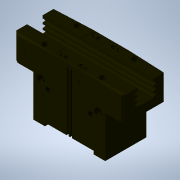
# Autodesk Inventor part: SCHUNK-5524256 Gehaeuse-PGN-plus-P 160-GKS
Saved by Autodesk Inventor 2021 (Build 250183000, 183)
## iProperties
Created: 2025-07-30
Part Number: SCHUNK-5524256 Gehaeuse-PGN-plus-P 160-GKS
Material: Generic
Catalog Web Link: www.cadenas.de
Description: Gehaeuse PGN-plus-P-2-finger parallel gripper
Vendor: SCHUNK
Document SubType Name: Modeling
Designer: psAdmin
Manufacturer: SCHUNK
Mass: 988.597 g
Surface Area: 1168.86 cm^2
Volume: 988.597 cm^3
Density: 1 g/cm^3
Appearance: PSOLRGB-128-128-0
Category: PARTsolutions
Company: SCHUNK
Title: SCHUNK-5524256 Gehaeuse-PGN-plus-P 160-GKS
Author: Cadenas PARTsolutions
Comments: 2-finger parallel gripper
PSOL_IDENT_0: {$CADENAS_DATA/23d-libs/schunk/greifsysteme/greifmodule/greifmodule_pneumatisch/2_finger_parallelgre
PSOL_IDENT_1: ifer/2_finger_universalgreifer/pgn_plus_p/pgnplus_p_geh.prj},238 {VTYP=3D},{NB=SCHUNK-5524256 Gehaeu
PSOL_IDENT_2: se-PGN-plus-P 160-GKS},{LINA=SCHUNK-5524256 Gehaeuse-PGN-plus-P 160-GKS},{NN=Gehaeuse PGN-plus-P},{D
PSOL_IDENT_3: ATE=24.02.2025 16:11:11},{GEOMDATE=14.02.2025 07:59:00},{VERSION=},{LINEID=170},{WBVAR=},{WBNUMERIC=
PSOL_IDENT_4: }  {NB=SCHUNK-5524256 Gehaeuse-PGN-plus-P 160-GKS},{LINA=SCHUNK-5524256 Gehaeuse-PGN-plus-P 160-GKS}
PSOL_IDENT_5: ,{KT=DUMMY},{IDNR=5524256},{TYP=PGN-plus-P 160-GKS},{TYP1=8.000},{TYP2=1.000},{L1=192.000},{B1=72.00
PSOL_IDENT_6: 0},{H1=116.000},{F1=3.500},{WF1=30.000},{L2=125.000},{H2=72.000},{BAVZ=27.390},{TAVZ=86.650},{L1VZ=4
PSOL_IDENT_7: .310},{L2VZ=8.500},{HVZ=5.235},{B1VZ=5.975},{B2VZ=3.170},{F2=0.500},{DNNHS=4.100},{BNNHS=3.400},{LNN
PSOL_IDENT_8: HS=106.600},{L1NNHS=3.000},{L2NNHS=34.100},{LS1=100.000},{LS2=56.000},{SD1=10.500},{ST1=55.500},{G1=
PSOL_IDENT_9: 8.000},{GT1=20.500},{KL1=6.800},{SD2=12.000},{ST2=3.900},{SD3=14.000},{ST3=20.000},{DB1=9.000},{LS3=
PSOL_IDENT_10: 100.000},{LS4=68.000},{B1A=56.000},{B2A=69.000},{RA=6.500},{TA=1.000},{L1TYP=92.000},{L2TYP=15.100},
PSOL_IDENT_11: {LTYP=64.300},{BTYP=16.300},{TTYP=0.700},{B3A=113.100},{B4A=85.100},{T2A=5.500},{R1A=7.450},{R2A=15.
PSOL_IDENT_12: 000},{G2=5.000},{LG1=111.500},{LG2=99.500},{TKT=1.500},{D1=1.000},{D2=0.500},{TT=1.800},{LB1=148.500
PSOL_IDENT_13: },{DB2=8.200},{TB2=86.350},{DB3=6.800},{LD1=0.000},{D3=0.000},{TD3=0.000},{L3=138.500},{H3=55.750},{
PSOL_IDENT_14: B2=20.000},{B3=61.325},{R1=35.000},{H4=30.000},{LG3=58.000},{LG4=74.000},{SD4=0.000},{ST4=0.000},{G3=
PSOL_IDENT_15: 5.000},{TKT2=1.500},{D4=1.000},{D5=0.500},{TT2=1.800},{G4=9.730},{GT4=7.000},{KT4=11.000},{LG5=58.00
PSOL_IDENT_16: 0},{LG6=74.000},{SDZHU=8.000},{TSZHU=2.900},{G5=5.000},{GT5=13.000},{KT5=15.500},{LS5=26.000},{LS6=5
PSOL_IDENT_17: 6.000},{SD5=7.000},{ST5=1.500},{G6=3.000},{GT6=6.000},{KT6=7.500},{SD6=5.000},{ST6=0.600},{LS7=43.00
PSOL_IDENT_18: 0},{LS8=56.000},{H5=50.000},{LG7=86.000},{LG8=45.000},{G7=4.000},{GT7=7.000},{KT7=10.000},{LG9=59.40
PSOL_IDENT_19: 0},{LG10=6.500},{LG11=66.900},{G8=3.000},{GT8=5.000},{KT8=8.000},{L1G=61.000},{HG=6.000},{LA=29.000}
PSOL_IDENT_20: ,{LB=24.000},{LKLH=6.5},{L1DYNFASE=56.000},{FDYNFASE=5.000},{BMMS=0.000},{TMMS=0.000},{LMMS=0.000},{
PSOL_IDENT_21: FASEDYN=0.500},{SLGD=5.0},{SLGT=4.0},{LAGD=5.0},{LAGT=4.0},{CNSCTN=}
NB: SCHUNK-5524256 Gehaeuse-PGN-plus-P 160-GKS
NN: Gehaeuse PGN-plus-P
NT: 2-finger parallel gripper
NBSYN: SCHUNK-$IDNR. Gehaeuse-$TYP.
LINA: SCHUNK-5524256 Gehaeuse-PGN-plus-P 160-GKS
CATALOG: SCHUNK
IDNR: 5524256
TYP: PGN-plus-P 160-GKS
TYP1: 8
TYP2: 1
L1: 192
B1: 72
H1: 116
F1: 3.5
WF1: 30
L2: 125
H2: 72
BAVZ: 27.39
TAVZ: 86.65
L1VZ: 4.31
L2VZ: 8.5
HVZ: 5.235
B1VZ: 5.975
B2VZ: 3.17
F2: 0.5
DNNHS: 4.1
BNNHS: 3.4
LNNHS: 106.6
L1NNHS: 3
L2NNHS: 34.1
LS1: 100
LS2: 56
SD1: 10.5
ST1: 55.5
G1: 8
GT1: 20.5
KL1: 6.8
SD2: 12
ST2: 3.9
SD3: 14
ST3: 20
DB1: 9
LS3: 100
LS4: 68
B1A: 56
B2A: 69
RA: 6.5
TA: 1
L1TYP: 92
L2TYP: 15.1
LTYP: 64.3
BTYP: 16.3
TTYP: 0.7
B3A: 113.1
B4A: 85.1
T2A: 5.5
R1A: 7.45
R2A: 15
G2: 5
LG1: 111.5
LG2: 99.5
TKT: 1.5
D1: 1
D2: 0.5
TT: 1.8
LB1: 148.5
DB2: 8.2
TB2: 86.35
DB3: 6.8
LD1: 0
D3: 0
TD3: 0
L3: 138.5
H3: 55.75
B2: 20
B3: 61.325
R1: 35
H4: 30
LG3: 58
LG4: 74
SD4: 0
ST4: 0
G3: 5
TKT2: 1.5
D4: 1
D5: 0.5
TT2: 1.8
G4: 9.73
GT4: 7
KT4: 11
LG5: 58
LG6: 74
SDZHU: 8
TSZHU: 2.9
G5: 5
GT5: 13
KT5: 15.5
LS5: 26
LS6: 56
SD5: 7
ST5: 1.5
G6: 3
GT6: 6
KT6: 7.5
SD6: 5
ST6: 0.6
LS7: 43
LS8: 56
H5: 50
LG7: 86
LG8: 45
G7: 4
GT7: 7
KT7: 10
LG9: 59.4
LG10: 6.5
LG11: 66.9
G8: 3
GT8: 5
KT8: 8
L1G: 61
HG: 6
LA: 29
LB: 24
L1DYNFASE: 56
FDYNFASE: 5
BMMS: 0
TMMS: 0
LMMS: 0
FASEDYN: 0.5
SLGD: 5
SLGT: 4
LAGD: 5
LAGT: 4
SUPPLIER: SCHUNK
ARTICLENO: SCHUNK-5524256 Gehaeuse-PGN-plus-P 160-GKS
BOMINFO: SCHUNK-5524256 Gehaeuse-PGN-plus-P 160-GKS
CREATOR: CADENAS GmbH
Autodesk Inventor part; units mm, degrees
ref_plane "YZ Plane" through (0, 0, 0) normal (1, 0, 0) x (0, 1, 0)
ref_plane "XZ Plane" through (0, 0, 0) normal (0, 1, 0) x (-1, 0, 0)
ref_plane "XY Plane" through (0, 0, 0) normal (0, 0, 1) x (1, 0, 0)
sketch "Sketch_1" plane through (0, 0, 0) normal (0, 1, 0) x (-1, 0, 0)
  line L0 (96, -32.5) -> (96, 32.5)
  line L1 (96, 32.5) -> (89.9378, 36)
  line L2 (89.9378, 36) -> (-89.9378, 36)
  line L3 (-89.9378, 36) -> (-96, 32.5)
  line L4 (-96, 32.5) -> (-96, -32.5)
  line L5 (-96, -32.5) -> (-89.9378, -36)
  line L6 (-89.9378, -36) -> (89.9378, -36)
  line L7 (89.9378, -36) -> (96, -32.5)
  constraints: 16 end point
extrude "Extrusion1" add sketch "Sketch_1" along normal blind 116
sketch "Sketch_2" plane through (0, 0, 0) normal (0, 0, 1) x (1, 0, 0)
  line L0 (62.5, 72) -> (62.5, 0)
  line L1 (62.5, 0) -> (96, 0)
  line L2 (96, 0) -> (96, 72)
  line L3 (96, 72) -> (62.5, 72)
  constraints: 8 end point
extrude "Extrusion2" cut sketch "Sketch_2" along normal mid plane 72
sketch "Sketch_3" plane through (0, 0, 0) normal (0, 0, 1) x (1, 0, 0)
  line L0 (-96, 0) -> (-62.5, 0)
  line L1 (-62.5, 0) -> (-62.5, 72)
  line L2 (-62.5, 72) -> (-96, 72)
  line L3 (-96, 72) -> (-96, 0)
  constraints: 8 end point
extrude "Extrusion3" cut sketch "Sketch_3" along normal mid plane 72
sketch "Sketch_4" plane through (0, 0, 0) normal (1, 0, 0) x (0, 1, 0)
  line L0 (116, 13.695) -> (86.65, 13.695)
  line L1 (86.65, 13.695) -> (86.65, -13.695)
  line L2 (86.65, -13.695) -> (116, -13.695)
  line L3 (116, -13.695) -> (116, 13.695)
  constraints: 8 end point
extrude "Extrusion4" cut sketch "Sketch_4" along normal mid plane 192
sketch "Sketch_5" plane through (0, 0, 0) normal (1, 0, 0) x (0, 1, 0)
  line L0 (92.3915, 18.93) -> (89.5285, 18.93)
  arc A0 (89.5285, 18.93) -> (89.3353, 18.7818) centre (89.5285, 18.73) ccw
  line L1 (89.3353, 18.7818) -> (88.0122, 13.8432)
  arc A1 (87.819, 13.695) -> (88.0122, 13.8432) centre (87.819, 13.895) ccw
  line L2 (87.819, 13.695) -> (94.101, 13.695)
  arc A2 (93.9078, 13.8432) -> (94.101, 13.695) centre (94.101, 13.895) ccw
  line L3 (93.9078, 13.8432) -> (92.5847, 18.7818)
  arc A3 (92.5847, 18.7818) -> (92.3915, 18.93) centre (92.3915, 18.73) ccw
  constraints: 8 end point, 8 point on circle, 4 centre point
extrude "Extrusion5" cut sketch "Sketch_5" along normal mid plane 192
pattern_linear "Rectangular Pattern1" count 3 spacing 8.5 along (0, 1, 0) of "Extrusion5"
sketch "Sketch_7" plane through (0, 0, 0) normal (1, 0, 0) x (0, 1, 0)
  line L0 (94.101, -13.695) -> (87.819, -13.695)
  arc A0 (88.0122, -13.8432) -> (87.819, -13.695) centre (87.819, -13.895) ccw
  line L1 (88.0122, -13.8432) -> (89.3353, -18.7818)
  arc A1 (89.3353, -18.7818) -> (89.5285, -18.93) centre (89.5285, -18.73) ccw
  line L2 (89.5285, -18.93) -> (92.3915, -18.93)
  arc A2 (92.3915, -18.93) -> (92.5847, -18.7818) centre (92.3915, -18.73) ccw
  line L3 (92.5847, -18.7818) -> (93.9078, -13.8432)
  arc A3 (94.101, -13.695) -> (93.9078, -13.8432) centre (94.101, -13.895) ccw
  constraints: 8 end point, 8 point on circle, 4 centre point
extrude "Extrusion6" cut sketch "Sketch_7" along normal mid plane 192
pattern_linear "Rectangular Pattern2" count 3 spacing 8.5 along (0, 1, 0) of "Extrusion6"
sketch "Sketch_9" plane through (0, 0, 0) normal (1, 0, 0) x (0, 1, 0)
  line L0 (116, -35.5) -> (115.5, -36)
  line L1 (115.5, -36) -> (116, -36)
  line L2 (116, -36) -> (116, -35.5)
  constraints: 6 end point
extrude "Extrusion7" cut sketch "Sketch_9" along normal mid plane 192
sketch "Sketch_10" plane through (0, 0, 0) normal (1, 0, 0) x (0, 1, 0)
  line L0 (116, 36) -> (115.5, 36)
  line L1 (115.5, 36) -> (116, 35.5)
  line L2 (116, 35.5) -> (116, 36)
  constraints: 6 end point
extrude "Extrusion8" cut sketch "Sketch_10" along normal mid plane 192
sketch "Sketch_36" plane through (28, 0, 0) normal (1, 0, 0) x (0, 0, -1)
  line L0 (-36, 116) -> (-36, 115.6464)
  line L1 (-36, 115.6464) -> (-35.6464, 116)
  line L2 (-35.6464, 116) -> (-36, 116)
  constraints: 6 end point
sketch "Sketch_93" plane through (96, 0, 0) normal (1, 0, 0) x (0, 0, -1)
  line L0 (-36, 116) -> (-36, 112.4645)
  line L1 (-36, 112.4645) -> (-32.4645, 116)
  line L2 (-32.4645, 116) -> (-36, 116)
  constraints: 6 end point
loft "Loft1" cut profiles "Sketch_36", "Sketch_93"
sketch "Sketch_94" plane through (-28, 0, 0) normal (1, 0, 0) x (0, 0, -1)
  line L0 (-36, 116) -> (-36, 115.6464)
  line L1 (-36, 115.6464) -> (-35.6464, 116)
  line L2 (-35.6464, 116) -> (-36, 116)
  constraints: 6 end point
sketch "Sketch_95" plane through (-96, 0, 0) normal (1, 0, 0) x (0, 0, -1)
  line L0 (-36, 116) -> (-36, 112.4645)
  line L1 (-36, 112.4645) -> (-32.4645, 116)
  line L2 (-32.4645, 116) -> (-36, 116)
  constraints: 6 end point
loft "Loft2" cut profiles "Sketch_95", "Sketch_94"
sketch "Sketch_96" plane through (28, 0, 0) normal (1, 0, 0) x (0, 0, -1)
  line L0 (36, 116) -> (35.6464, 116)
  line L1 (35.6464, 116) -> (36, 115.6464)
  line L2 (36, 115.6464) -> (36, 116)
  constraints: 6 end point
sketch "Sketch_97" plane through (96, 0, 0) normal (1, 0, 0) x (0, 0, -1)
  line L0 (36, 116) -> (32.4645, 116)
  line L1 (32.4645, 116) -> (36, 112.4645)
  line L2 (36, 112.4645) -> (36, 116)
  constraints: 6 end point
loft "Loft3" cut profiles "Sketch_96", "Sketch_97"
sketch "Sketch_98" plane through (-28, 0, 0) normal (1, 0, 0) x (0, 0, -1)
  line L0 (36, 116) -> (35.6464, 116)
  line L1 (35.6464, 116) -> (36, 115.6464)
  line L2 (36, 115.6464) -> (36, 116)
  constraints: 6 end point
sketch "Sketch_99" plane through (-96, 0, 0) normal (1, 0, 0) x (0, 0, -1)
  line L0 (36, 116) -> (32.4645, 116)
  line L1 (32.4645, 116) -> (36, 112.4645)
  line L2 (36, 112.4645) -> (36, 116)
  constraints: 6 end point
loft "Loft4" cut profiles "Sketch_99", "Sketch_98"
sketch "Sketch_11" plane through (0, 0, 0) normal (0, 1, 0) x (-1, 0, 0)
  arc A0 (-4.7, 35.2456) -> (-1.3, 35.2456) centre (-3, 34.1) ccw
  line L0 (-1.3, 35.2456) -> (-1.3, 37)
  line L1 (-1.3, 37) -> (-4.7, 37)
  line L2 (-4.7, 37) -> (-4.7, 35.2456)
  constraints: 6 end point, 2 point on circle, 1 centre point
extrude "Extrusion9" cut sketch "Sketch_11" along normal blind 106.6
pattern_linear "Rectangular Pattern3" count 2 spacing 6 along (-1, 0, 0) of "Extrusion9"
sketch "Sketch_13" plane through (0, 0, 36) normal (0, 0, 1) x (1, 0, 0)
  circle A0 centre (3, 106.6) radius 1.7
  constraints: 1 centre point
extrude "Extrusion10" cut sketch "Sketch_13" against normal blind 2.05
pattern_linear "Rectangular Pattern4" count 2 spacing 6 along (-1, 0, 0) of "Extrusion10"
sketch "Sketch_15" plane through (0, 106.6, 0) normal (0, 1, 0) x (1, 0, 0)
  line L0 (3, -100) -> (3, 100)
  arc A0 (3, -36.15) -> (3, -32.05) centre (3, -34.1) ccw
  line L1 (3, -36.15) -> (3, -32.05)
  constraints: 4 end point, 2 point on circle, 1 centre point
revolve "Revolution1" cut sketch "Sketch_15" angle 360 about axis through (3, 106.6, 100) along (0, 0, 1)
pattern_linear "Rectangular Pattern5" count 2 spacing 6 along (-1, 0, 0) of "Revolution1"
sketch "Sketch_17" plane through (50, 0, 0) normal (1, 0, 0) x (0, 0, -1)
  line L0 (28, 0) -> (28, 116)
  line L1 (28, 116) -> (33.25, 116)
  line L2 (33.25, 116) -> (33.25, 60.5)
  line L3 (33.25, 60.5) -> (31.3235, 60.5)
  line L4 (31.3235, 60.5) -> (31.3235, 0)
  line L5 (31.3235, 0) -> (28, 0)
  line L6 (28, 0) -> (28, 116)
  constraints: 14 end point
revolve "Revolution2" cut sketch "Sketch_17" angle 360 about axis through (50, 0, -28) along (0, -1, 0)
thread "Thread1" size "M8x1.25" class "6H" standard "ISO Metric profile" length 20.5
pattern_linear "Rectangular Pattern6" count 2 spacing 114.6124 along (-0.872506, 0, 0.4886034) of "Revolution2"
sketch "Sketch_108" plane through (50, 0, 0) normal (1, 0, 0) x (0, 0, -1)
  line L0 (28, 0) -> (28, 116)
  line L1 (28, 116) -> (31.4, 116)
  line L2 (31.4, 116) -> (31.4, 0)
  line L3 (31.4, 0) -> (28, 0)
  line L4 (28, 0) -> (28, 116)
  constraints: 10 end point
revolve "Revolution3" cut sketch "Sketch_108" angle 360 about axis through (50, 0, -28) along (0, -1, 0)
pattern_linear "Rectangular Pattern7" count 2 spacing 114.6124 along (-0.872506, 0, 0.4886034) of "Revolution3"
sketch "Sketch_19" plane through (50, 0, 0) normal (1, 0, 0) x (0, 0, -1)
  line L0 (-28, 0) -> (-28, 116)
  line L1 (-28, 116) -> (-22.75, 116)
  line L2 (-22.75, 116) -> (-22.75, 60.5)
  line L3 (-22.75, 60.5) -> (-24.6765, 60.5)
  line L4 (-24.6765, 60.5) -> (-24.6765, 3.9)
  line L5 (-24.6765, 3.9) -> (-22, 3.9)
  line L6 (-22, 3.9) -> (-22, 0)
  line L7 (-22, 0) -> (-28, 0)
  line L8 (-28, 0) -> (-28, 116)
  constraints: 18 end point
revolve "Revolution4" cut sketch "Sketch_19" angle 360 about axis through (50, 0, 28) along (0, -1, 0)
thread "Thread2" size "M8x1.25" class "6H" standard "ISO Metric profile" length 16.6
pattern_linear "Rectangular Pattern8" count 2 spacing 114.6124 along (-0.872506, 0, -0.4886034) of "Revolution4"
sketch "Sketch_110" plane through (50, 0, 0) normal (1, 0, 0) x (0, 0, -1)
  line L0 (-28, 0) -> (-28, 116)
  line L1 (-28, 116) -> (-24.6, 116)
  line L2 (-24.6, 116) -> (-24.6, 0)
  line L3 (-24.6, 0) -> (-28, 0)
  line L4 (-28, 0) -> (-28, 116)
  constraints: 10 end point
revolve "Revolution5" cut sketch "Sketch_110" angle 360 about axis through (50, 0, 28) along (0, -1, 0)
pattern_linear "Rectangular Pattern9" count 2 spacing 114.6124 along (-0.872506, 0, -0.4886034) of "Revolution5"
sketch "Sketch_21" plane through (50, 0, 0) normal (1, 0, 0) x (0, 0, -1)
  line L0 (36, 68) -> (-36, 68)
  line L1 (-36, 68) -> (-36, 75)
  line L2 (-36, 75) -> (-16, 75)
  line L3 (-16, 75) -> (-16, 72.5)
  line L4 (-16, 72.5) -> (32.1, 72.5)
  line L5 (32.1, 72.5) -> (32.1, 74)
  line L6 (32.1, 74) -> (36, 74)
  line L7 (36, 74) -> (36, 68)
  line L8 (36, 68) -> (-36, 68)
  constraints: 18 end point
revolve "Revolution6" cut sketch "Sketch_21" angle 360 about axis through (50, 68, -36) along (0, 0, -1)
pattern_linear "Rectangular Pattern10" count 2 spacing 100 along (-1, 0, 0) of "Revolution6"
sketch "Sketch_23" plane through (0, 116, 0) normal (0, 1, 0) x (1, 0, 0)
  line L0 (-28, 28) -> (-28, -28)
  arc A0 (-28, -28) -> (-21.5, -34.5) centre (-21.5, -28) ccw
  line L1 (-21.5, -34.5) -> (21.5, -34.5)
  arc A1 (21.5, -34.5) -> (28, -28) centre (21.5, -28) ccw
  line L2 (28, -28) -> (28, 28)
  arc A2 (28, 28) -> (21.5, 34.5) centre (21.5, 28) ccw
  line L3 (21.5, 34.5) -> (-21.5, 34.5)
  arc A3 (-21.5, 34.5) -> (-28, 28) centre (-21.5, 28) ccw
  constraints: 8 end point, 8 point on circle, 4 centre point
extrude "Extrusion11" cut sketch "Sketch_23" against normal blind 1
sketch "Sketch_24" plane through (0, 0, 36) normal (0, 0, 1) x (1, 0, 0)
  arc A0 (23.25, 108.3) -> (23.25, 92) centre (23.25, 100.15) ccw
  line L0 (23.25, 92) -> (71.25, 92)
  arc A1 (71.25, 92) -> (71.25, 108.3) centre (71.25, 100.15) ccw
  line L1 (71.25, 108.3) -> (23.25, 108.3)
  constraints: 4 end point, 4 point on circle, 2 centre point
extrude "Extrusion12" cut sketch "Sketch_24" against normal blind 0.7
sketch "Sketch_70" plane through (0, 0, 36) normal (0, 0, 1) x (1, 0, 0)
  arc A0 (-71.25, 108.3) -> (-71.25, 92) centre (-71.25, 100.15) ccw
  line L0 (-71.25, 92) -> (-23.25, 92)
  arc A1 (-23.25, 92) -> (-23.25, 108.3) centre (-23.25, 100.15) ccw
  line L1 (-23.25, 108.3) -> (-71.25, 108.3)
  constraints: 4 end point, 4 point on circle, 2 centre point
extrude "Extrusion13" cut sketch "Sketch_70" against normal blind 0.7
sketch "Sketch_58" plane through (0, 0, 0) normal (0, 1, 0) x (-1, 0, 0)
  line L0 (56.55, -7.201) -> (56.55, 7.201)
  arc A0 (56.55, 7.201) -> (47.1959, 21.0979) centre (41.55, 7.201) ccw
  arc A1 (42.55, 28) -> (47.1959, 21.0979) centre (50, 28) ccw
  line L1 (42.55, 28) -> (42.55, 38)
  line L2 (42.55, 38) -> (-42.55, 38)
  line L3 (-42.55, 38) -> (-42.55, 28)
  arc A2 (-47.1959, 21.0979) -> (-42.55, 28) centre (-50, 28) ccw
  arc A3 (-47.1959, 21.0979) -> (-56.55, 7.201) centre (-41.55, 7.201) ccw
  line L4 (-56.55, 7.201) -> (-56.55, -7.201)
  arc A4 (-56.55, -7.201) -> (-47.1959, -21.0979) centre (-41.55, -7.201) ccw
  arc A5 (-42.55, -28) -> (-47.1959, -21.0979) centre (-50, -28) ccw
  line L5 (-42.55, -28) -> (-42.55, -36)
  line L6 (-42.55, -36) -> (42.55, -36)
  line L7 (42.55, -36) -> (42.55, -28)
  arc A6 (47.1959, -21.0979) -> (42.55, -28) centre (50, -28) ccw
  arc A7 (47.1959, -21.0979) -> (56.55, -7.201) centre (41.55, -7.201) ccw
  constraints: 16 end point, 16 point on circle, 8 centre point
extrude "Extrusion14" cut sketch "Sketch_58" along normal blind 5.5
sketch "Sketch_45" plane through (0, 0, 0) normal (1, 0, 0) x (0, 1, 0)
  line L0 (86, -35.9) -> (86, -36)
  line L1 (86, -36) -> (116, -36)
  line L2 (116, -36) -> (116, -35.9)
  line L3 (116, -35.9) -> (86, -35.9)
  constraints: 8 end point
extrude "Extrusion15" cut sketch "Sketch_45" along normal mid plane 192
sketch "Sketch_54" plane through (0, 0, 0) normal (1, 0, 0) x (0, 1, 0)
  line L0 (50, -35.9) -> (0, -35.9)
  line L1 (0, -35.9) -> (0, -36)
  line L2 (0, -36) -> (50, -36)
  line L3 (50, -36) -> (50, -35.9)
  constraints: 8 end point
extrude "Extrusion16" cut sketch "Sketch_54" along normal mid plane 192
sketch "Sketch_27" plane through (0, 0, 0) normal (1, 0, 0) x (0, 1, 0)
  line L0 (111.5, 35.9) -> (111.5, 36)
  line L1 (111.5, 36) -> (114, 36)
  line L2 (114, 36) -> (114, 35.6)
  line L3 (114, 35.6) -> (113.7, 35.9)
  line L4 (113.7, 35.9) -> (111.5, 35.9)
  line L5 (111.5, 35.9) -> (111.5, 36)
  constraints: 12 end point
revolve "Revolution7" cut sketch "Sketch_27" angle 360 about axis through (0, 111.5, 35.9) along (0, 0, -1)
sketch "Sketch_28" plane through (0, 0, 0) normal (1, 0, 0) x (0, 1, 0)
  line L0 (99.5, -35.9) -> (99.5, -35.8)
  line L1 (99.5, -35.8) -> (101.7, -35.8)
  line L2 (101.7, -35.8) -> (102, -35.5)
  line L3 (102, -35.5) -> (102, -35.9)
  line L4 (102, -35.9) -> (99.5, -35.9)
  line L5 (99.5, -35.9) -> (99.5, -35.8)
  constraints: 12 end point
revolve "Revolution8" cut sketch "Sketch_28" angle 360 about axis through (0, 99.5, -35.9) along (0, 0, -1)
sketch "Sketch_29" plane through (0, 111.5, 35.9) normal (0, 0, 1) x (0, 1, 0)
  arc A0 (-1, 0.866) -> (-1.25, 0.433) centre (-1.125, 0.6495) ccw
  arc A1 (-1.25, -0.433) -> (-1.25, 0.433) centre (-1.5, 0) ccw
  arc A2 (-1.25, -0.433) -> (-1, -0.866) centre (-1.125, -0.6495) ccw
  arc A3 (-0.25, -1.299) -> (-1, -0.866) centre (-0.75, -1.299) ccw
  arc A4 (-0.25, -1.299) -> (0.25, -1.299) centre (0, -1.299) ccw
  arc A5 (1, -0.866) -> (0.25, -1.299) centre (0.75, -1.299) ccw
  arc A6 (1, -0.866) -> (1.25, -0.433) centre (1.125, -0.6495) ccw
  arc A7 (1.25, 0.433) -> (1.25, -0.433) centre (1.5, 0) ccw
  arc A8 (1.25, 0.433) -> (1, 0.866) centre (1.125, 0.6495) ccw
  arc A9 (0.25, 1.299) -> (1, 0.866) centre (0.75, 1.299) ccw
  arc A10 (0.25, 1.299) -> (-0.25, 1.299) centre (0, 1.299) ccw
  arc A11 (-1, 0.866) -> (-0.25, 1.299) centre (-0.75, 1.299) ccw
  constraints: 24 point on circle, 12 centre point
extrude "Extrusion17" cut sketch "Sketch_29" against normal blind 1.8
sketch "Sketch_30" plane through (0, 99.5, -35.8) normal (0, 0, -1) x (0, 1, 0)
  arc A0 (-1, 0.866) -> (-1.25, 0.433) centre (-1.125, 0.6495) ccw
  arc A1 (-1.25, -0.433) -> (-1.25, 0.433) centre (-1.5, 0) ccw
  arc A2 (-1.25, -0.433) -> (-1, -0.866) centre (-1.125, -0.6495) ccw
  arc A3 (-0.25, -1.299) -> (-1, -0.866) centre (-0.75, -1.299) ccw
  arc A4 (-0.25, -1.299) -> (0.25, -1.299) centre (0, -1.299) ccw
  arc A5 (1, -0.866) -> (0.25, -1.299) centre (0.75, -1.299) ccw
  arc A6 (1, -0.866) -> (1.25, -0.433) centre (1.125, -0.6495) ccw
  arc A7 (1.25, 0.433) -> (1.25, -0.433) centre (1.5, 0) ccw
  arc A8 (1.25, 0.433) -> (1, 0.866) centre (1.125, 0.6495) ccw
  arc A9 (0.25, 1.299) -> (1, 0.866) centre (0.75, 1.299) ccw
  arc A10 (0.25, 1.299) -> (-0.25, 1.299) centre (0, 1.299) ccw
  arc A11 (-1, 0.866) -> (-0.25, 1.299) centre (-0.75, 1.299) ccw
  constraints: 24 point on circle, 12 centre point
extrude "Extrusion18" cut sketch "Sketch_30" against normal blind 1.8
sketch "Sketch_31" plane through (0, 0, 0) normal (0, 0, 1) x (1, 0, 0)
  line L0 (74.25, 0) -> (74.25, 86.65)
  line L1 (74.25, 86.65) -> (77.65, 86.65)
  line L2 (77.65, 86.65) -> (77.65, 86.35)
  line L3 (77.65, 86.35) -> (78.35, 86.35)
  line L4 (78.35, 86.35) -> (78.35, 0)
  line L5 (78.35, 0) -> (74.25, 0)
  line L6 (74.25, 0) -> (74.25, 86.65)
  constraints: 14 end point
revolve "Revolution9" cut sketch "Sketch_31" angle 360 about axis through (74.25, 0, 0) along (0, -1, 0)
pattern_linear "Rectangular Pattern11" count 2 spacing 148.5 along (-1, 0, 0) of "Revolution9"
sketch "Sketch_35" plane through (0, 55.75, 0) normal (0, 1, 0) x (1, 0, 0)
  line L0 (62.5, 30.6625) -> (62.5, -30.6625)
  arc A0 (69.25, -10) -> (62.5, -30.6625) centre (97.5, -30.6625) ccw
  line L1 (69.25, -10) -> (69.25, 10)
  arc A1 (62.5, 30.6625) -> (69.25, 10) centre (97.5, 30.6625) ccw
  constraints: 4 end point, 4 point on circle, 2 centre point
extrude "Extrusion19" add sketch "Sketch_35" along normal blind 16.25
sketch "Sketch_92" plane through (0, 55.75, 0) normal (0, 1, 0) x (1, 0, 0)
  line L0 (-69.25, 10) -> (-69.25, -10)
  arc A0 (-62.5, -30.6625) -> (-69.25, -10) centre (-97.5, -30.6625) ccw
  line L1 (-62.5, -30.6625) -> (-62.5, 30.6625)
  arc A1 (-69.25, 10) -> (-62.5, 30.6625) centre (-97.5, 30.6625) ccw
  constraints: 4 end point, 4 point on circle, 2 centre point
extrude "Extrusion20" add sketch "Sketch_92" along normal blind 16.25
sketch "Sketch_87" plane through (0, 58, 0) normal (0, 1, 0) x (1, 0, 0)
  line L0 (37, 35.95) -> (37, 36.1)
  line L1 (37, 36.1) -> (39.5, 36.1)
  line L2 (39.5, 36.1) -> (39.5, 35.75)
  line L3 (39.5, 35.75) -> (39.3, 35.95)
  line L4 (39.3, 35.95) -> (37, 35.95)
  line L5 (37, 35.95) -> (37, 36.1)
  constraints: 12 end point
revolve "Revolution10" cut sketch "Sketch_87" angle 360 about axis through (37, 58, -35.95) along (0, 0, 1)
sketch "Pattern_24_SKETCH_1" plane through (0, 58, 0) normal (0, 1, 0) x (1, 0, 0)
  line L0 (-37, 35.85) -> (-37, 36)
  line L1 (-37, 36) -> (-34.5, 36)
  line L2 (-34.5, 36) -> (-34.5, 35.65)
  line L3 (-34.5, 35.65) -> (-34.7, 35.85)
  line L4 (-34.7, 35.85) -> (-37, 35.85)
  line L5 (-37, 35.85) -> (-37, 36)
  constraints: 12 end point
revolve "Revolution11" cut sketch "Pattern_24_SKETCH_1" angle 360 about axis through (-37, 58, -35.85) along (0, 0, 1)
sketch "Sketch_89" plane through (37, 58, -35.95) normal (0, 0, -1) x (1, 0, 0)
  arc A0 (-1, 0.866) -> (-1.25, 0.433) centre (-1.125, 0.6495) ccw
  arc A1 (-1.25, -0.433) -> (-1.25, 0.433) centre (-1.5, 0) ccw
  arc A2 (-1.25, -0.433) -> (-1, -0.866) centre (-1.125, -0.6495) ccw
  arc A3 (-0.25, -1.299) -> (-1, -0.866) centre (-0.75, -1.299) ccw
  arc A4 (-0.25, -1.299) -> (0.25, -1.299) centre (0, -1.299) ccw
  arc A5 (1, -0.866) -> (0.25, -1.299) centre (0.75, -1.299) ccw
  arc A6 (1, -0.866) -> (1.25, -0.433) centre (1.125, -0.6495) ccw
  arc A7 (1.25, 0.433) -> (1.25, -0.433) centre (1.5, 0) ccw
  arc A8 (1.25, 0.433) -> (1, 0.866) centre (1.125, 0.6495) ccw
  arc A9 (0.25, 1.299) -> (1, 0.866) centre (0.75, 1.299) ccw
  arc A10 (0.25, 1.299) -> (-0.25, 1.299) centre (0, 1.299) ccw
  arc A11 (-1, 0.866) -> (-0.25, 1.299) centre (-0.75, 1.299) ccw
  constraints: 24 point on circle, 12 centre point
extrude "Extrusion21" cut sketch "Sketch_89" against normal blind 1.8
pattern_linear "Rectangular Pattern12" count 2 spacing 74 along (-1, 0, 0) of "Extrusion21"
sketch "Sketch41" plane through (62.5, 72, 36) normal (0, 0, 1) x (1, 0, 0)
  point P0 (-25.5, -14)
hole "Hole1" at (37, 58, 36) direction (0, 0, -1) diameter 8 depth 11.3497 tip angle 118 taper from width 8.4473 to width 7.985 over 7.4 thread size "Rc 1/8" standard "ISO Taper Internal"
pattern_linear "Rectangular Pattern13" count 2 spacing 74 along (-1, 0, 0) of "Hole1"
sketch "Sketch42" plane through (0, 115, 0) normal (0, 1, 0) x (1, 0, 0)
  point P0 (13, 28)
hole "Hole2" at (13, 115, -28) direction (0, -1, 0) diameter 4.134 depth 18.6602 tip angle 118 counterbore diameter 8 counterbore depth 2.9 thread size "M5x0.8" class "6H" standard "ISO Metric profile"
pattern_linear "Rectangular Pattern14" count 2 spacing 26 along (-1, 0, 0) count 2 spacing 56 along (0, 0, 1) of "Hole2"
sketch "Sketch_52" plane through (21.5, 0, 0) normal (1, 0, 0) x (0, 0, -1)
  line L0 (28, 105.0987) -> (28, 115)
  line L1 (28, 115) -> (31.5, 115)
  line L2 (31.5, 115) -> (31.5, 114.4)
  line L3 (31.5, 114.4) -> (30.7121, 114.4)
  line L4 (30.7121, 114.4) -> (30.5, 114.1879)
  line L5 (30.5, 114.1879) -> (30.5, 113.5)
  line L6 (30.5, 113.5) -> (29.2295, 113.0376)
  line L7 (29.2295, 113.0376) -> (29.2295, 105.8375)
  line L8 (29.2295, 105.8375) -> (28, 105.0987)
  line L9 (28, 105.0987) -> (28, 115)
  constraints: 20 end point
revolve "Revolution12" cut sketch "Sketch_52" angle 360 about axis through (21.5, 105.0987, -28) along (0, -1, 0)
thread "Thread3" size "M3x0.5" class "6H" standard "ISO Metric profile" length 5.9016
pattern_linear "Rectangular Pattern15" count 2 spacing 43 along (-1, 0, 0) count 2 spacing 56 along (0, 0, 1) of "Revolution12"
sketch "Sketch44" plane through (-96, 72, -32.5) normal (-1, 0, 0) x (0, 0, 1)
  point P0 (10, 14)
hole "Hole3" at (-96, 86, -22.5) direction (1, 0, 0) diameter 3.242 depth 10.2277 tip angle 118 thread size "M4x0.7" class "6H" standard "ISO Metric profile"
pattern_linear "Rectangular Pattern16" count 2 spacing 45 along (0, 0, 1) of "Hole3"
sketch "Sketch45" plane through (96, 72, 32.5) normal (1, 0, 0) x (0, 0, -1)
  point P0 (55, 14)
hole "Hole4" at (96, 86, -22.5) direction (-1, 0, 0) diameter 3.242 depth 10.2277 tip angle 118 thread size "M4x0.7" class "6H" standard "ISO Metric profile"
pattern_linear "Rectangular Pattern17" count 2 spacing 45 along (0, 0, 1) of "Hole4"
sketch "Sketch46" plane through (-69.25, 55.75, -10) normal (-1, 0, 0) x (0, 0, 1)
  point P0 (3.5, 3.65)
hole "Hole5" at (-69.25, 59.4, -6.5) direction (1, 0, 0) diameter 2.459 depth 8.1625 tip angle 118 thread size "M3x0.5" class "6H" standard "ISO Metric profile"
pattern_linear "Rectangular Pattern18" count 2 spacing 7.5 along (0, 1, 0) of "Hole5"
sketch "Sketch47" plane through (69.25, 55.75, 10) normal (1, 0, 0) x (0, 0, -1)
  point P0 (16.5, 3.65)
hole "Hole6" at (69.25, 59.4, -6.5) direction (-1, 0, 0) diameter 2.459 depth 8.1625 tip angle 118 thread size "M3x0.5" class "6H" standard "ISO Metric profile"
pattern_linear "Rectangular Pattern19" count 2 spacing 7.5 along (0, 1, 0) of "Hole6"
sketch "Sketch_67" plane through (0, 0, 36) normal (0, 0, 1) x (1, 0, 0)
  line L0 (23.9996, 61) -> (26, 55)
  line L1 (26, 55) -> (26.9996, 55)
  line L2 (26.9996, 55) -> (29, 61)
  line L3 (29, 61) -> (28.25, 61)
  line L4 (28.25, 61) -> (27.7496, 59.4688)
  line L5 (27.7496, 59.4688) -> (25.25, 59.4688)
  line L6 (25.25, 59.4688) -> (24.7496, 61)
  line L7 (24.7496, 61) -> (23.9996, 61)
  line L8 (25.3748, 58.9576) -> (26.5004, 55.5112)
  line L9 (26.5004, 55.5112) -> (27.6248, 58.9576)
  line L10 (27.6248, 58.9576) -> (25.3748, 58.9576)
  constraints: 22 end point
extrude "Extrusion22" cut sketch "Sketch_67" against normal blind 0.2
sketch "Sketch_68" plane through (0, 0, 36) normal (0, 0, 1) x (1, 0, 0)
  line L0 (-28.6248, 59.596) -> (-28.6248, 58.9576)
  line L1 (-28.6248, 58.9576) -> (-28.5, 58.5748)
  line L2 (-28.5, 58.5748) -> (-28.1244, 58.0648)
  line L3 (-28.1244, 58.0648) -> (-27.8748, 57.9364)
  line L4 (-27.8748, 57.9364) -> (-28.1244, 57.8092)
  line L5 (-28.1244, 57.8092) -> (-28.5, 57.298)
  line L6 (-28.5, 57.298) -> (-28.6248, 56.9152)
  line L7 (-28.6248, 56.9152) -> (-28.6248, 56.4052)
  line L8 (-28.6248, 56.4052) -> (-28.5, 56.0212)
  line L9 (-28.5, 56.0212) -> (-28.1244, 55.5112)
  line L10 (-28.1244, 55.5112) -> (-27.6252, 55.1284)
  line L11 (-27.6252, 55.1284) -> (-27, 55)
  line L12 (-27, 55) -> (-24, 55)
  line L13 (-24, 55) -> (-24, 61)
  line L14 (-24, 61) -> (-27, 61)
  line L15 (-27, 61) -> (-27.6252, 60.8728)
  line L16 (-27.6252, 60.8728) -> (-28.1244, 60.49)
  line L17 (-28.1244, 60.49) -> (-28.5, 59.9788)
  line L18 (-28.5, 59.9788) -> (-28.6248, 59.596)
  line L19 (-27.8748, 59.4688) -> (-27.8748, 59.086)
  line L20 (-27.8748, 59.086) -> (-27.75, 58.702)
  line L21 (-27.75, 58.702) -> (-27.5004, 58.4476)
  line L22 (-27.5004, 58.4476) -> (-27.1248, 58.3192)
  line L23 (-27.1248, 58.3192) -> (-24.75, 58.3192)
  line L24 (-24.75, 58.3192) -> (-24.75, 60.2344)
  line L25 (-24.75, 60.2344) -> (-27.1248, 60.2344)
  line L26 (-27.1248, 60.2344) -> (-27.5004, 60.1072)
  line L27 (-27.5004, 60.1072) -> (-27.75, 59.8516)
  line L28 (-27.75, 59.8516) -> (-27.8748, 59.4688)
  line L29 (-27.8748, 56.5324) -> (-27.75, 56.1496)
  line L30 (-27.75, 56.1496) -> (-27.5004, 55.894)
  line L31 (-27.5004, 55.894) -> (-27.1248, 55.7668)
  line L32 (-27.1248, 55.7668) -> (-24.75, 55.7668)
  line L33 (-24.75, 55.7668) -> (-24.75, 57.5536)
  line L34 (-24.75, 57.5536) -> (-27.1248, 57.5536)
  line L35 (-27.1248, 57.5536) -> (-27.5004, 57.4264)
  line L36 (-27.5004, 57.4264) -> (-27.75, 57.1708)
  line L37 (-27.75, 57.1708) -> (-27.8748, 56.788)
  line L38 (-27.8748, 56.788) -> (-27.8748, 56.5324)
  constraints: 78 end point
extrude "Extrusion23" cut sketch "Sketch_68" against normal blind 0.2
ref_plane "ANS_1_XY" through (3, 0, 34.1) normal (0, 1, 0) x (1, 0, 0)
ref_plane "ANS_1_YZ" through (3, 0, 34.1) normal (1, 0, 0) x (0, 0, -1)
ref_plane "ANS_1_ZX" through (3, 0, 34.1) normal (0, 0, -1) x (0, 1, 0)
ref_plane "IP_IN_XY" through (74.25, 86.35, 0) normal (0, 1, 0) x (1, 0, 0)
ref_plane "IP_IN_YZ" through (74.25, 86.35, 0) normal (1, 0, 0) x (0, 0, -1)
ref_plane "IP_IN_ZX" through (74.25, 86.35, 0) normal (0, 0, -1) x (0, 1, 0)
ref_plane "IP_IN2_XY" through (-74.25, 86.35, 0) normal (0, 1, 0) x (1, 0, 0)
ref_plane "IP_IN2_YZ" through (-74.25, 86.35, 0) normal (1, 0, 0) x (0, 0, -1)
ref_plane "IP_IN2_ZX" through (-74.25, 86.35, 0) normal (0, 0, -1) x (0, 1, 0)
ref_plane "TYP2_XY" through (-47.25, 100.15, 35.3) normal (0, 0, 1) x (1, 0, 0)
ref_plane "TYP2_YZ" through (-47.25, 100.15, 35.3) normal (1, 0, 0) x (0, 1, 0)
ref_plane "TYP2_ZX" through (-47.25, 100.15, 35.3) normal (0, 1, 0) x (0, 0, 1)
ref_plane "Typ_XY" through (47.25, 100.15, 35.3) normal (0, 0, 1) x (1, 0, 0)
ref_plane "Typ_YZ" through (47.25, 100.15, 35.3) normal (1, 0, 0) x (0, 1, 0)
ref_plane "Typ_ZX" through (47.25, 100.15, 35.3) normal (0, 1, 0) x (0, 0, 1)
ref_plane "adb_XY" through (0, 115, 0) normal (0, 1, 0) x (1, 0, 0)
ref_plane "adb_YZ" through (0, 115, 0) normal (1, 0, 0) x (0, 0, -1)
ref_plane "adb_ZX" through (0, 115, 0) normal (0, 0, -1) x (0, 1, 0)
ref_plane "adb_sd_XY" through (0, 116, 0) normal (0, 1, 0) x (1, 0, 0)
ref_plane "adb_sd_YZ" through (0, 116, 0) normal (1, 0, 0) x (0, 0, -1)
ref_plane "adb_sd_ZX" through (0, 116, 0) normal (0, 0, -1) x (0, 1, 0)
ref_plane "dec_XY" through (0, 5.5, 0) normal (0, 1, 0) x (1, 0, 0)
ref_plane "dec_YZ" through (0, 5.5, 0) normal (1, 0, 0) x (0, 0, -1)
ref_plane "dec_ZX" through (0, 5.5, 0) normal (0, 0, -1) x (0, 1, 0)
ref_plane "einbau_XY" through (0, 0, 0) normal (0, 1, 0) x (1, 0, 0)
ref_plane "einbau_YZ" through (0, 0, 0) normal (1, 0, 0) x (0, 0, -1)
ref_plane "einbau_ZX" through (0, 0, 0) normal (0, 0, -1) x (0, 1, 0)
ref_plane "klh_1_XY" through (-69.25, 59.4, -6.5) normal (1, 0, 0) x (0, 0, -1)
ref_plane "klh_1_YZ" through (-69.25, 59.4, -6.5) normal (0, 0, -1) x (0, 1, 0)
ref_plane "klh_1_ZX" through (-69.25, 59.4, -6.5) normal (0, 1, 0) x (1, 0, 0)
ref_plane "klh_2_XY" through (69.25, 59.4, -6.5) normal (1, 0, 0) x (0, 0, -1)
ref_plane "klh_2_YZ" through (69.25, 59.4, -6.5) normal (0, 0, -1) x (0, 1, 0)
ref_plane "klh_2_ZX" through (69.25, 59.4, -6.5) normal (0, 1, 0) x (1, 0, 0)
ref_plane "klh_3_XY" through (-69.25, 66.9, -6.5) normal (1, 0, 0) x (0, 0, -1)
ref_plane "klh_3_YZ" through (-69.25, 66.9, -6.5) normal (0, 0, -1) x (0, 1, 0)
ref_plane "klh_3_ZX" through (-69.25, 66.9, -6.5) normal (0, 1, 0) x (1, 0, 0)
ref_plane "klh_4_XY" through (69.25, 66.9, -6.5) normal (1, 0, 0) x (0, 0, -1)
ref_plane "klh_4_YZ" through (69.25, 66.9, -6.5) normal (0, 0, -1) x (0, 1, 0)
ref_plane "klh_4_ZX" through (69.25, 66.9, -6.5) normal (0, 1, 0) x (1, 0, 0)
ref_plane "zhu_1_XY" through (50, 3.9, 28) normal (0, 1, 0) x (1, 0, 0)
ref_plane "zhu_1_YZ" through (50, 3.9, 28) normal (1, 0, 0) x (0, 0, -1)
ref_plane "zhu_1_ZX" through (50, 3.9, 28) normal (0, 0, -1) x (0, 1, 0)
ref_plane "zhu_2_XY" through (-50, 3.9, -28) normal (0, 1, 0) x (1, 0, 0)
ref_plane "zhu_2_YZ" through (-50, 3.9, -28) normal (1, 0, 0) x (0, 0, -1)
ref_plane "zhu_2_ZX" through (-50, 3.9, -28) normal (0, 0, -1) x (0, 1, 0)
ref_plane "zhu_3_XY" through (50, 68, -32.1) normal (0, 0, 1) x (1, 0, 0)
ref_plane "zhu_3_YZ" through (50, 68, -32.1) normal (1, 0, 0) x (0, 1, 0)
ref_plane "zhu_3_ZX" through (50, 68, -32.1) normal (0, 1, 0) x (0, 0, 1)
ref_plane "zhu_4_XY" through (-50, 68, -32.1) normal (0, 0, 1) x (1, 0, 0)
ref_plane "zhu_4_YZ" through (-50, 68, -32.1) normal (1, 0, 0) x (0, 1, 0)
ref_plane "zhu_4_ZX" through (-50, 68, -32.1) normal (0, 1, 0) x (0, 0, 1)
body "Solid1"
